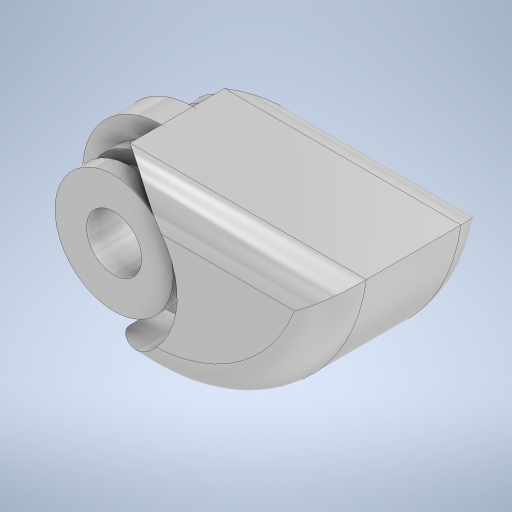
# Autodesk Inventor part: TapPart
Saved by Autodesk Inventor 2024 (Build 280153000, 153)
## iProperties
Created: 2024-03-20
Part Number: TapPart
Material: Generic
Document SubType Name: Modeling
Designer: Wojtek
Density: 1 g/cm^3
Appearance: Default
Author: Wojtek
Autodesk Inventor part; units mm, degrees
ref_plane "YZ Plane" through (0, 0, 0) normal (1, 0, 0) x (0, 1, 0)
ref_plane "XZ Plane" through (0, 0, 0) normal (0, 1, 0) x (-1, 0, 0)
ref_plane "XY Plane" through (0, 0, 0) normal (0, 0, 1) x (1, 0, 0)
sketch "Sketch1" plane through (0, 0, 0) normal (0, 0, 1) x (1, 0, 0)
  circle A0 centre (0, 0) radius 10
  line L0 (0, 10) -> (30, 10)
  arc A1 (0, -10) -> (30, 10) centre (6.2119, 13.1822) ccw
  circle A2 centre (0, 0) radius 3.5
  circle A3 centre (0, 0) radius 7.5
  circle A4 centre (0, 0) radius 6
  dimension "d0" = 20
  dimension "d1" = 30
  dimension "d2" = 24
  dimension "d3" = 10
  dimension "d4" = 13.1822
  dimension "d5" = 7
  dimension "d6" = 15
  dimension "d7" = 12
  constraints: 5 centre point, 4 coincident, 4 point on circle, 2 end point, 1 horizontal
  measures "d0" diameter of A0
  measures "d1" distance of L0.start L0.end
  measures "d2" radius of A1
  measures "d3" distance from line of point (0, 0) L0
  measures "d4" vertical distance of point (0, 0) A1.centre
  measures "d5" diameter of A2
  measures "d6" diameter of A3
  measures "d7" diameter of A4
extrude "Extrusion1" add sketch "Sketch1" along normal mid plane 20 contours A0 L0 A1
extrude "Extrusion2" add sketch "Sketch1" along normal mid plane 4 contours A0 | A3 | A4
extrude "Extrusion3" add sketch "Sketch1" along normal mid plane 8 contours A3 | A4
extrude "Extrusion4" add sketch "Sketch1" along normal mid plane 12 contours A4
sketch "Sketch2" plane through (0, 0, 6) normal (0, 0, 1) x (1, 0, 0)
  circle A0 centre (0, 0) radius 7.5
  circle A1 centre (0, 0) radius 3.5
  dimension "d16" = 15
  dimension "d18" = 7
  constraints: 2 centre point, 2 coincident
  measures "d16" diameter of A0
  measures "d18" diameter of A1
sketch "Sketch3" plane through (0, 0, -6) normal (0, 0, -1) x (-1, 0, 0)
  circle A0 centre (0, 0) radius 7.5
  circle A1 centre (0, 0) radius 3.5
  dimension "d17" = 15
  dimension "d19" = 7
  constraints: 2 centre point, 2 coincident
  measures "d17" diameter of A0
  measures "d19" diameter of A1
extrude "Extrusion5" add sketch "Sketch3" along normal blind 2
extrude "Extrusion6" add sketch "Sketch2" along normal blind 2
fillet "Fillet1" radius 4 4 edges at (15, 10, -10) (19.5247, -6.7871, -10) (19.5247, -6.7871, 10) (15, 10, 10)
